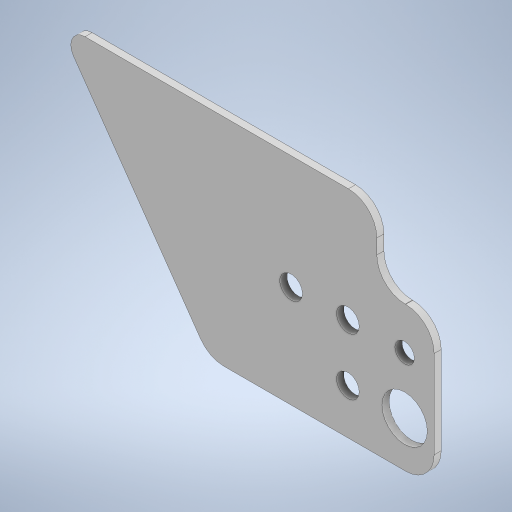
# Autodesk Inventor part: Sleds poly V4
Saved by Autodesk Inventor 2023 (Build 270158000, 158)
## iProperties
Created: 2024-01-30
Part Number: Sleds poly V4
Material: Generic
Document SubType Name: Modeling
Designer: Robodox
Density: 1 g/cm^3
Appearance: Default
Author: Robodox
Autodesk Inventor part; units mm, degrees
ref_plane "YZ Plane" through (0, 0, 0) normal (1, 0, 0) x (0, 1, 0)
ref_plane "XZ Plane" through (0, 0, 0) normal (0, 1, 0) x (-1, 0, 0)
ref_plane "XY Plane" through (0, 0, 0) normal (0, 0, 1) x (1, 0, 0)
sketch "Sketch1" plane through (0, 0, 0) normal (0, 0, 1) x (1, 0, 0)
  line L0 (47.6451, -34.29) -> (92.334, -34.29)
  line L1 (47.6451, -34.29) -> (41.1035, -34.29)
  line L2 (39.8575, 12.7612) -> (31.599, 12.7612)
  line L3 (39.8575, 12.7612) -> (20.8075, 12.7612)
  line L4 (79.512, 12.7612) -> (37.4294, 12.7612)
  line L5 (79.512, -31.9773) -> (79.512, 12.7612)
  line L6 (92.334, -18.8499) -> (92.334, 1.5256)
  line L7 (92.334, -18.8499) -> (92.334, -34.29)
  circle A0 centre (85.7451, -25.4) radius 3.9624
  circle A1 centre (85.7451, -12.7) radius 2.1844
  circle A2 centre (73.0451, -12.7) radius 2.54
  circle A3 centre (60.3451, -12.7) radius 2.54
  circle A4 centre (73.0451, -25.4) radius 2.54
  line L8 (-341.1851, -3.2325) -> (91.1147, -3.2325)
  line L9 (25.7365, 2.0147) -> (20.8075, 12.7612)
  line L10 (91.1147, -3.2325) -> (92.334, -3.2325)
  circle A5 centre (85.7451, -25.4) radius 5.08
  line L11 (39.8575, 12.7612) -> (8.1075, 12.7612)
  line L12 (8.1075, 12.7612) -> (56.4583, -56.2272)
  line L13 (41.1035, -35.5589) -> (41.9728, -35.5589)
  line L14 (41.9728, -35.5589) -> (92.334, -35.5589)
  line L15 (92.334, -35.5589) -> (92.334, -34.29)
  point P0 (0, 0)
  point P1 (0, 0)
  point P2 (41.3274, -31.9773)
  point P3 (79.512, -18.8499)
  point P4 (79.512, -3.2325)
  point P5 (79.512, -3.2325)
  dimension "d0" = 19.05
  dimension "d1" = 432.2999
  dimension "d2" = 10.16
  dimension "d3" = 31.75
  constraints: 32 end point, 8 point on line, 6 centre point, 4 horizontal, 2 perpendicular, 1 coincident, 1 parallel, 1 vertical
  measures "d0" distance of L2.start L3.end
  measures "d1" distance of L8.start L8.end
  measures "d2" diameter of A5
  measures "d3" distance of L2.start L11.end
extrude "Extrusion1" add sketch "Sketch1" along normal blind 1.5875 contours L4 L5 L8 L12 L11 L3 L2 | L8 L10 L6 L7 L15 L14 L12
fillet "Fillet1" radius 6.35 5 edges at (79.512, 12.7612, 0.7937) (79.512, -3.2325, 0.7937) (92.334, -3.2325, 0.7937) (92.334, -35.5589, 0.7937) (41.9728, -35.5589, 0.7937)
fillet "Fillet2" radius 3.175 1 edges at (8.1075, 12.7612, 0.7937)
body "Solid1"
